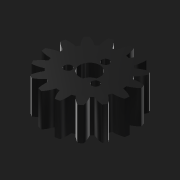
# Autodesk Inventor part: Spur Gear13
Saved by Autodesk Inventor 2017 (Build 210142000, 142)
## iProperties
Created: 2018-10-09
Part Number: Spur Gear13
Material: ABS Plastic
Document SubType Name: Modeling
Designer: Zach
Categories: <?xml version="1.0" encoding="UTF-16"?> <MemberInstance><Categories><FamilyTemplate><FamilyTemplateParameter ValueType="xs:double" Id="1" ObjectReferenceKey="da_z" ObjectType="kUserParameterObject"/><FamilyTemplateParameter ValueType="xs:double" Id="2" ObjectReferenceKey="da_b" ObjectType="kUserParameterObject"/><FamilyTemplateParameter ValueType="xs:double" Id="3" ObjectReferenceKey="da_beta" ObjectType="kUserParameterObject"/><FamilyTemplateParameter ValueType="xs:double" Id="4" ObjectReferenceKey="da_da" ObjectType="kUserParameterObject"/><FamilyTemplateParameter ValueType="xs:double" Id="5" ObjectReferenceKey="da_aw" ObjectType="kUserParameterObject"/><FamilyTemplateParameter ValueType="xs:string" Id="6" ObjectReferenceKey="EAIAABAAAACIAQAAAAAAAIAAAAAAAAAA" ObjectType="83910656" SubObjectId="SurfaceGeometry"/></FamilyTemplate><ParamToTemplateMap><ParamToTemplate CategoryParameter="//CategoryParameter[@InternalName='046C89C9-8512-4d59-83FE-43B91F4F132A']" TemplateParameter="1"/><ParamToTemplate CategoryParameter="//CategoryParameter[@InternalName='2552DF32-E462-4b46-AEBF-C6C7768E72AC']" TemplateParameter="2"/><ParamToTemplate CategoryParameter="//CategoryParameter[@InternalName='C9EE641D-15FC-4fae-A226-E94C4372FDD7']" TemplateParameter="3"/><ParamToTemplate><ParamToTemplate CategoryParameter="//CategoryParameter[@InternalName='00B6519A-459B-49c7-AD84-2E56D39A5744']" ConstantValue="0.000000"/></ParamToTemplate><ParamToTemplate><ParamToTemplate CategoryParameter="//CategoryParameter[@InternalName='04B31F0E-C7A6-4894-AA32-9629BEFACF47']" ConstantValue="1.000000"/></ParamToTemplate><ParamToTemplate><ParamToTemplate CategoryParameter="//CategoryParameter[@InternalName='43CBEC2E-7847-49e7-A936-2F7889FCB2D9']" ConstantValue="0.250000"/></ParamToTemplate><ParamToTemplate><ParamToTemplate CategoryParameter="//CategoryParameter[@InternalName='B1EFC894-105D-4ebd-86BF-FA20ED196853']" ConstantValue="0.350000"/></ParamToTemplate><ParamToTemplate><ParamToTemplate CategoryParameter="//CategoryParameter[@InternalName='51175063-3D10-4879-93E8-6246FE8B403D']" ConstantValue="2060000000.000000"/></ParamToTemplate><ParamToTemplate><ParamToTemplate CategoryParameter="//CategoryParameter[@InternalName='A3A52E27-4454-46a9-B0BD-C932399B70AF']" ConstantValue="0.300000"/></ParamToTemplate><ParamToTemplate><ParamToTemplate CategoryParameter="//CategoryParameter[@InternalName='91B76062-C214-41d9-B1B9-14D2AB99603D']" ConstantValue="0.200000"/></ParamToTemplate><ParamToTemplate><ParamToTemplate CategoryParameter="//CategoryParameter[@InternalName='374E806E-8B8A-4dda-A9AA-1039D6500AD2']" ConstantValue="5.000000"/></ParamToTemplate><ParamToTemplate><ParamToTemplate CategoryParameter="//CategoryParameter[@InternalName='2D373A89-B862-43d6-8D0B-0CBF12AB9F6C']" ConstantValue="0.392699"/></ParamToTemplate><ParamToTemplate CategoryParameter="//CategoryParameter[@InternalName='37777632-D6A2-4fac-9D53-DB8ACD95C989']" TemplateParameter="4"/><ParamToTemplate CategoryParameter="//CategoryParameter[@InternalName='FD1017F1-B727-4f7e-9707-0F86F1FF9423']" TemplateParameter="5"/><ParamToTemplate><ParamToTemplate CategoryParameter="//CategoryParameter[@InternalName='9E1B4470-B2D3-4ff1-B813-535BB4CDF51A']" ConstantValue="3520000.000000"/></ParamToTemplate><ParamToTemplate><ParamToTemplate CategoryParameter="//CategoryParameter[@InternalName='F8452263-BFF6-458c-9FB1-07C4B99E95CD']" ConstantValue="11400000.000000"/></ParamToTemplate><ParamToTemplate><ParamToTemplate CategoryParameter="//CategoryParameter[@InternalName='3E3BB259-FD49-497f-8171-6EBC954A3479']" ConstantValue="2.000000"/></ParamToTemplate><ParamToTemplate CategoryParameter="//CategoryParameter[@InternalName='27C3BAF2-7550-4e4b-AE2C-0DB134B7D9B7']" TemplateParameter="6"/></ParamToTemplateMap><Category DisplayName="Gear" InternalName="DC85795E-93AB-48d5-8EEE-5A27447B64BD" Mnemonic="Gear"><CategoryParameter DisplayName="z" InternalName="046C89C9-8512-4d59-83FE-43B91F4F132A" Mnemonic="z"/><CategoryParameter DisplayName="b" InternalName="2552DF32-E462-4b46-AEBF-C6C7768E72AC" Mnemonic="b"/><CategoryParameter DisplayName="||b|" InternalName="C9EE641D-15FC-4fae-A226-E94C4372FDD7" Mnemonic="beta"/><CategoryParameter DisplayName="x" InternalName="00B6519A-459B-49c7-AD84-2E56D39A5744" Mnemonic="x"/><CategoryParameter DisplayName="a*" InternalName="04B31F0E-C7A6-4894-AA32-9629BEFACF47" Mnemonic="a"/><CategoryParameter DisplayName="c*" InternalName="43CBEC2E-7847-49e7-A936-2F7889FCB2D9" Mnemonic="c"/><CategoryParameter DisplayName="r|.f|*" InternalName="B1EFC894-105D-4ebd-86BF-FA20ED196853" Mnemonic="rf"/><CategoryParameter DisplayName="E" InternalName="51175063-3D10-4879-93E8-6246FE8B403D" Mnemonic="E"/><CategoryParameter DisplayName="||m|" InternalName="A3A52E27-4454-46a9-B0BD-C932399B70AF" Mnemonic="mi"/><Category DisplayName="SpurGear" InternalName="26C5A22E-A91E-4dfd-A3B3-23CCAFAE1764" Mnemonic="SpurGear"><CategoryParameter DisplayName="m" InternalName="91B76062-C214-41d9-B1B9-14D2AB99603D" Mnemonic="m"/><CategoryParameter DisplayName="P" InternalName="374E806E-8B8A-4dda-A9AA-1039D6500AD2" Mnemonic="PP"/><CategoryParameter DisplayName="||a|" InternalName="2D373A89-B862-43d6-8D0B-0CBF12AB9F6C" Mnemonic="alpha"/><CategoryParameter DisplayName="d|.a|" InternalName="37777632-D6A2-4fac-9D53-DB8ACD95C989" Mnemonic="da"/><CategoryParameter DisplayName="a|.w|" InternalName="FD1017F1-B727-4f7e-9707-0F86F1FF9423" Mnemonic="aw"/><CategoryParameter DisplayName="||s||.Flim|" InternalName="9E1B4470-B2D3-4ff1-B813-535BB4CDF51A" Mnemonic="sFlim"/><CategoryParameter DisplayName="||s||.Hlim|" InternalName="F8452263-BFF6-458c-9FB1-07C4B99E95CD" Mnemonic="sHlim"/><CategoryParameter DisplayName="type" InternalName="3E3BB259-FD49-497f-8171-6EBC954A3479" Mnemonic="type"/><CategoryParameter DisplayName="PitchDiameter" InternalName="27C3BAF2-7550-4e4b-AE2C-0DB134B7D9B7" Mnemonic="IDS_PITCHDIAM"/></Category></Category></Categories></MemberInstance>
Density: 1.06 g/cm^3
Appearance: Smooth - Black
Mass: 7.97468 g
Surface Area: 42.1284 cm^2
Volume: 7.52328 cm^3
CustomPartVersion: 1
Author: Zach
Autodesk Inventor part; units mm, degrees
ref_plane "YZ Plane" through (0, 0, 0) normal (1, 0, 0) x (0, 1, 0)
ref_plane "XZ Plane" through (0, 0, 0) normal (0, 1, 0) x (-1, 0, 0)
ref_plane "XY Plane" through (0, 0, 0) normal (0, 0, 1) x (1, 0, 0)
sketch "Sketch1" plane through (0, 0, 0) normal (0, 0, 1) x (1, 0, 0)
  circle A0 centre (0, 0) radius 16.5
  dimension "d0" = 33
  constraints: 1 centre point
  measures "d0" diameter of A0
extrude "Extrusion1" add sketch "Sketch1" along normal blind 20
ref_plane "Work Plane2" through (0, 0, 10) normal (0, 0, 1) x (1, 0, 0)
sketch "Sketch2" plane through (0, 0, 0) normal (0, 0, -1) x (-1, 0, 0)
  circle A0 centre (0, 0) radius 16.5 projected
  circle A1 centre (0, 0) radius 15
  dimension "d3" = 30
  constraints: 1 centre point, 1 coincident
  measures "d3" diameter of A1
surface extrude "Pitch Diameter" sketch "Sketch2" against normal through all shown no curves A1
ref_plane "Work Plane8" through (0, 0, 0) normal (0.9781476, 0.2079117, 0) x (0, 0, 1)
ref_plane "Work Plane9" through (0, 0, 0) normal (1, 0, 0) x (0, 1, 0)
spur gear teeth "Spur Gear" teeth 15 pitch diameter 30 tip diameter 33 root diameter 25 face width 20 start plane through (0, 0, 0) normal (0, 0, -1) x (-1, 0, 0)
sketch "Sketch3" plane through (0, 0, 20) normal (0, 0, 1) x (1, 0, 0)
  circle A0 centre (0, 0) radius 4
  dimension "d49" = 8
  constraints: 1 centre point, 1 coincident
  measures "d49" diameter of A0
extrude "Extrusion2" cut sketch "Sketch3" against normal through all
sketch "Sketch4" plane through (0, 0, 20) normal (0, 0, 1) x (1, 0, 0)
  circle A0 centre (0, 0) radius 12
  dimension "d52" = 24
  constraints: 1 centre point, 1 coincident
  measures "d52" diameter of A0
extrude "Extrusion3" cut sketch "Sketch4" against normal blind 12.7
sketch "Sketch5" plane through (0, 0, 0) normal (0, 0, -1) x (-1, 0, 0)
  circle A0 centre (0, 6.2) radius 1.5
  circle A1 centre (5.3694, -3.1) radius 1.5
  circle A2 centre (-5.3694, -3.1) radius 1.5
  point P0 (0, 0)
  dimension "d55" = 3
  dimension "d56" = 6.2
  dimension "d59" = 360
  constraints: 3 centre point, 1 vertical alignment, 7 other
  measures "d55" diameter of A0
  measures "d56" distance of A0.centre point (0, 0)
extrude "Extrusion4" cut sketch "Sketch5" against normal through all
sketch "Sketch6" plane through (0, 0, 0) normal (0, 0, -1) x (-1, 0, 0)
  circle A0 centre (0, 6.2) radius 1.5 projected
  circle A1 centre (0, 6.2) radius 4
  circle A2 centre (-5.3694, -3.1) radius 4
  circle A3 centre (5.3694, -3.1) radius 4
  point P0 (0, 0)
  dimension "d63" = 8
  dimension "d66" = 360
  constraints: 3 centre point, 1 coincident, 7 other
  measures "d63" diameter of A1
extrude "Extrusion5" cut sketch "Sketch6" against normal blind 3 contours A0 | A1 | A2 | A3
sketch "Sketch7" plane through (0, 0, 7.3) normal (0, 0, 1) x (1, 0, 0)
  circle A0 centre (0, 0) radius 22.5
  dimension "d70" = 45
  constraints: 1 centre point, 1 coincident
  measures "d70" diameter of A0
extrude "Extrusion6" cut sketch "Sketch7" along normal through all
sketch "Sketch9" plane through (0, 0, 7.3) normal (0, 0, 1) x (1, 0, 0)
  arc A0 (-1.9554, 12.3461) -> (-3.2352, 12.0741) centre (0, 0) ccw projected
  arc A1 (-3.2352, 12.0741) -> (-5.9131, 15.4041) centre (-14.1022, 6.077) ccw projected
  arc A2 (-5.9131, 15.4041) -> (-7.4908, 14.7016) centre (0, 0) ccw projected
  arc A3 (-7.4908, 14.7016) -> (-6.808, 10.4834) centre (4.9201, 14.5463) ccw projected
  arc A4 (-6.808, 10.4834) -> (-7.8665, 9.7143) centre (0, 0) ccw projected
  arc A5 (-7.8665, 9.7143) -> (-11.6673, 11.6673) centre (-15.3548, -0.1843) ccw projected
  arc A6 (-11.6673, 11.6673) -> (-12.8229, 10.3838) centre (0, 0) ccw projected
  arc A7 (-12.8229, 10.3838) -> (-10.4834, 6.808) centre (-1.4218, 15.2899) ccw projected
  arc A8 (-10.4834, 6.808) -> (-11.1376, 5.6749) centre (0, 0) ccw projected
  arc A9 (-11.1376, 5.6749) -> (-15.4041, 5.9131) centre (-13.9524, -6.4137) ccw projected
  arc A10 (-15.4041, 5.9131) -> (-15.9378, 4.2705) centre (0, 0) ccw projected
  arc A11 (-15.9378, 4.2705) -> (-12.3461, 1.9554) centre (-7.5178, 13.3898) ccw projected
  arc A12 (-12.3461, 1.9554) -> (-12.4829, 0.6542) centre (0, 0) ccw projected
  arc A13 (-12.4829, 0.6542) -> (-16.4774, -0.8635) centre (-10.1374, -11.5341) ccw projected
  arc A14 (-16.4774, -0.8635) -> (-16.2969, -2.5812) centre (0, 0) ccw projected
  arc A15 (-16.2969, -2.5812) -> (-12.0741, -3.2352) centre (-12.314, 9.1744) ccw projected
  arc A16 (-12.0741, -3.2352) -> (-11.6698, -4.4796) centre (0, 0) ccw projected
  arc A17 (-11.6698, -4.4796) -> (-14.7016, -7.4908) centre (-4.5697, -14.6602) ccw projected
  arc A18 (-14.7016, -7.4908) -> (-13.8381, -8.9865) centre (0, 0) ccw projected
  arc A19 (-13.8381, -8.9865) -> (-9.7143, -7.8665) centre (-14.9809, 3.3727) ccw projected
  arc A20 (-9.7143, -7.8665) -> (-8.8388, -8.8388) centre (0, 0) ccw projected
  arc A21 (-8.8388, -8.8388) -> (-10.3838, -12.8229) centre (1.7883, -15.2514) ccw projected
  arc A22 (-10.3838, -12.8229) -> (-8.9865, -13.8381) centre (0, 0) ccw projected
  arc A23 (-8.9865, -13.8381) -> (-5.6749, -11.1376) centre (-15.0576, -3.0122) ccw projected
  arc A24 (-5.6749, -11.1376) -> (-4.4796, -11.6698) centre (0, 0) ccw projected
  arc A25 (-4.4796, -11.6698) -> (-4.2705, -15.9378) centre (7.837, -13.2055) ccw projected
  arc A26 (-4.2705, -15.9378) -> (-2.5812, -16.2969) centre (0, 0) ccw projected
  arc A27 (-2.5812, -16.2969) -> (-0.6542, -12.4829) centre (-12.5306, -8.8763) ccw projected
  arc A28 (-0.6542, -12.4829) -> (0.6542, -12.4829) centre (0, 0) ccw projected
  arc A29 (0.6542, -12.4829) -> (2.5812, -16.2969) centre (12.5306, -8.8763) ccw projected
  arc A30 (2.5812, -16.2969) -> (4.2705, -15.9378) centre (0, 0) ccw projected
  arc A31 (4.2705, -15.9378) -> (4.4796, -11.6698) centre (-7.837, -13.2055) ccw projected
  arc A32 (4.4796, -11.6698) -> (5.6749, -11.1376) centre (0, 0) ccw projected
  arc A33 (5.6749, -11.1376) -> (8.9865, -13.8381) centre (15.0576, -3.0122) ccw projected
  arc A34 (8.9865, -13.8381) -> (10.3838, -12.8229) centre (0, 0) ccw projected
  arc A35 (10.3838, -12.8229) -> (8.8388, -8.8388) centre (-1.7883, -15.2514) ccw projected
  arc A36 (8.8388, -8.8388) -> (9.7143, -7.8665) centre (0, 0) ccw projected
  arc A37 (9.7143, -7.8665) -> (13.8381, -8.9865) centre (14.9809, 3.3727) ccw projected
  arc A38 (13.8381, -8.9865) -> (14.7016, -7.4908) centre (0, 0) ccw projected
  arc A39 (14.7016, -7.4908) -> (11.6698, -4.4796) centre (4.5697, -14.6602) ccw projected
  arc A40 (11.6698, -4.4796) -> (12.0741, -3.2352) centre (0, 0) ccw projected
  arc A41 (12.0741, -3.2352) -> (16.2969, -2.5812) centre (12.314, 9.1744) ccw projected
  arc A42 (16.2969, -2.5812) -> (16.4774, -0.8635) centre (0, 0) ccw projected
  arc A43 (16.4774, -0.8635) -> (12.4829, 0.6542) centre (10.1374, -11.5341) ccw projected
  arc A44 (12.4829, 0.6542) -> (12.3461, 1.9554) centre (0, 0) ccw projected
  arc A45 (12.3461, 1.9554) -> (15.9378, 4.2705) centre (7.5178, 13.3898) ccw projected
  arc A46 (15.9378, 4.2705) -> (15.4041, 5.9131) centre (0, 0) ccw projected
  arc A47 (15.4041, 5.9131) -> (11.1376, 5.6749) centre (13.9524, -6.4137) ccw projected
  arc A48 (11.1376, 5.6749) -> (10.4834, 6.808) centre (0, 0) ccw projected
  arc A49 (10.4834, 6.808) -> (12.8229, 10.3838) centre (1.4218, 15.2899) ccw projected
  arc A50 (12.8229, 10.3838) -> (11.6673, 11.6673) centre (0, 0) ccw projected
  arc A51 (11.6673, 11.6673) -> (7.8665, 9.7143) centre (15.3548, -0.1843) ccw projected
  arc A52 (7.8665, 9.7143) -> (6.808, 10.4834) centre (0, 0) ccw projected
  arc A53 (6.808, 10.4834) -> (7.4908, 14.7016) centre (-4.9201, 14.5463) ccw projected
  arc A54 (7.4908, 14.7016) -> (5.9131, 15.4041) centre (0, 0) ccw projected
  arc A55 (5.9131, 15.4041) -> (3.2352, 12.0741) centre (14.1022, 6.077) ccw projected
  arc A56 (3.2352, 12.0741) -> (1.9554, 12.3461) centre (0, 0) ccw projected
  arc A57 (1.9554, 12.3461) -> (0.8635, 16.4774) centre (-10.4113, 11.2875) ccw projected
  arc A58 (0.8635, 16.4774) -> (-0.8635, 16.4774) centre (0, 0) ccw projected
  arc A59 (-0.8635, 16.4774) -> (-1.9554, 12.3461) centre (10.4113, 11.2875) ccw projected
  circle A60 centre (-5.3694, -3.1) radius 1.5 projected
  circle A61 centre (0, 6.2) radius 1.5 projected
  circle A62 centre (5.3694, -3.1) radius 1.5 projected
  circle A63 centre (0, 0) radius 4 projected
extrude "Extrusion7" add sketch "Sketch9" along normal blind 5.7
sketch "Sketch11" plane through (0, 0, 0) normal (0, 0, -1) x (-1, 0, 0)
  circle A0 centre (0, 0) radius 4 projected
  point P0 (2.5812, -16.2969)
extrude "Extrusion9" add sketch "Sketch11" against normal blind 8
sketch "Sketch12" plane through (0, 0, 3) normal (0, 0, -1) x (-1, 0, 0)
  arc A0 (-3.9486, 0.6392) -> (-1.4208, -3.7392) centre (0, 0) ccw projected
  arc A1 (-3.9486, 0.6392) -> (-1.4208, -3.7392) centre (-5.3694, -3.1) ccw projected
  circle A2 centre (-5.3694, -3.1) radius 1.5 projected
  arc A3 (2.5278, 3.1) -> (-2.5278, 3.1) centre (0, 0) ccw projected
  arc A4 (2.5278, 3.1) -> (-2.5278, 3.1) centre (0, 6.2) ccw projected
  circle A5 centre (0, 6.2) radius 1.5 projected
  arc A6 (1.4208, -3.7392) -> (3.9486, 0.6392) centre (0, 0) ccw projected
  arc A7 (1.4208, -3.7392) -> (3.9486, 0.6392) centre (5.3694, -3.1) ccw projected
  circle A8 centre (5.3694, -3.1) radius 1.5 projected
  circle A9 centre (5.3694, -3.1) radius 4
  circle A10 centre (-5.3694, -3.1) radius 1.5 projected
  circle A11 centre (-5.3694, -3.1) radius 4
  circle A12 centre (0, 6.2) radius 1.5 projected
  circle A13 centre (0, 6.2) radius 4
  constraints: 3 coincident, 9 other
extrude "Extrusion10" cut sketch "Sketch12" along normal through all
equation "\"d0\" = da_da"
equation "\"d1\" = da_b"
equation "\"d3\" = da_dw"
equation "\"da_da\" = 33"
equation "\"da_b\" = 20"
equation "\"da_dw\" = 30"
body "Solid1"
body "Srf1"
